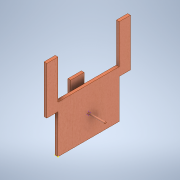
# Autodesk Inventor part: part1 edited
Saved by Autodesk Inventor 2021 (Build 250183000, 183)
## iProperties
Created: 2021-07-07
Part Number: part1 edited
Material: Wood (Walnut)
Document SubType Name: Modeling
Designer: VK
Density: 0.55 g/cm^3
Appearance: Walnut - Natural Polished
Author: VK
Autodesk Inventor part; units mm, degrees
ref_plane "YZ Plane" through (0, 0, 0) normal (1, 0, 0) x (0, 1, 0)
ref_plane "XZ Plane" through (0, 0, 0) normal (0, 1, 0) x (-1, 0, 0)
ref_plane "XY Plane" through (0, 0, 0) normal (0, 0, 1) x (1, 0, 0)
sketch "Sketch1" plane through (0, 0, 0) normal (1, 0, 0) x (0, 1, 0)
  line L0 (0, 0) -> (0, -110)
  line L1 (0, 0) -> (110, 0) construction
  line L2 (0, -110) -> (70, -110)
  line L3 (0, -110) -> (70, -110) construction
  line L4 (70, -110) -> (70, -130)
  line L5 (70, -130) -> (155, -130)
  line L6 (70, -130) -> (155, -130) construction
  line L7 (155, -130) -> (155, -110)
  line L8 (155, -110) -> (85, -110)
  line L9 (85, -110) -> (85, 0)
  line L10 (85, 0) -> (155, 0)
  line L11 (155, 0) -> (155, 20)
  line L12 (155, 20) -> (70, 20)
  line L13 (70, 20) -> (70, 0)
  line L14 (70, 0) -> (0, 0)
  dimension "d0" = 110
  dimension "d1" = 90
  dimension "d2" = 70
  dimension "d3" = 0
  dimension "d4" = 20
  dimension "d5" = 85
  dimension "d6" = 0
  dimension "d7" = 20
  dimension "d8" = 70
  dimension "d9" = 110
  dimension "d10" = 90
  dimension "d11" = 70
  dimension "d12" = 90
  dimension "d13" = 20
  dimension "d14" = 90
  dimension "d15" = 85
  dimension "d16" = 90
  constraints: 30 end point, 6 horizontal, 6 perpendicular, 3 equal length, 2 vertical, 1 collinear, 1 point on line
  measures "d0" distance of L0.start L0.end
  measures "d1" angle of L0 L1
  measures "d2" distance of L0.end L2.end
  measures "d3" distance between parallel lines of L2 L3
  measures "d4" distance of L2.end L4.end
  measures "d5" distance of L4.end L5.end
  measures "d6" distance between parallel lines of L5 L6
  measures "d7" distance of L6.end L7.end
  measures "d8" distance of L7.end L8.end
  measures "d9" distance of L8.end L9.end
  measures "d10" angle of L8 L9
  measures "d11" distance of L9.end L10.end
  measures "d12" angle of L9 L10
  measures "d13" distance of L10.end L11.end
  measures "d14" angle of L11 L10
  measures "d15" distance of L11.end L12.end
  measures "d16" angle of L12 L11
extrude "Extrusion1" add sketch "Sketch1" along normal blind 5
sketch "Sketch2" plane through (5, 0, 0) normal (1, 0, 0) x (0, 0, -1)
  point P0 (0, 0)
  point P1 (55, 40)
sketch "Sketch3" plane through (5, 0, 0) normal (1, 0, 0) x (0, 0, -1)
  circle A0 centre (55, 40) radius 1.5
  point P0 (0, 0)
  dimension "d19" = 3
  constraints: 1 centre point
  measures "d19" diameter of A0
extrude "Extrusion2" add sketch "Sketch3" along normal blind 30
sketch "Sketch4" plane through (0, 0, 0) normal (-1, 0, 0) x (0, 0, 1)
  line L0 (-67, 42.5) -> (-43, 42.5)
  line L1 (-43, 42.5) -> (-43, 37.5)
  line L2 (-43, 37.5) -> (-67, 37.5)
  line L3 (-67, 37.5) -> (-67, 42.5)
  circle A0 centre (-55, 40) radius 1.5 projected
  line L4 (-67, 42.5) -> (-43, 37.5) construction
  line L5 (-43, 42.5) -> (-67, 37.5) construction
  point P0 (0, 0)
  dimension "d22" = 24
  dimension "d23" = 5
  constraints: 12 end point, 2 midpoint, 2 parallel, 1 horizontal, 1 perpendicular
  measures "d22" distance of L1.end L2.end
  measures "d23" distance of L0.end L1.end
sketch "Sketch5" plane through (0, 0, 0) normal (-1, 0, 0) x (0, 0, 1)
  point P0 (0, 0)
sketch "Sketch6" plane through (0, 0, 0) normal (-1, 0, 0) x (0, 0, 1)
  circle A0 centre (-55, 40) radius 1.5
  point P0 (0, 0)
  constraints: 1 centre point
extrude "Extrusion3" add sketch "Sketch4" along normal blind 20 contours L0 L1 L2 L3 | A0
sketch "Sketch7" plane through (0, 42.5, -43) normal (0, 1, 0) x (1, 0, 0)
  line L0 (-20, 24) -> (-20, 0) projected
  line L1 (0, 24) -> (-20, 24) projected
  line L2 (-20, 0) -> (-15, 0)
  line L3 (-15, 0) -> (-15, 24)
  line L4 (-15, 24) -> (-20, 24)
  line L5 (-20, 24) -> (-20, 0)
  point P0 (0, -43)
  dimension "d26" = 5
  constraints: 8 end point, 2 parallel, 1 horizontal, 1 perpendicular, 1 point on line
  measures "d26" distance of L4.end L3.end
extrude "Extrusion4" add sketch "Sketch7" along normal blind 45
sketch "Sketch9" plane through (5, 0, 0) normal (1, 0, 0) x (0, 0, -1)
  point P0 (0, 0)
body "Solid1"
